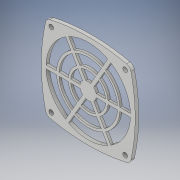
# Autodesk Inventor part: Speaker_Secure
Saved by Autodesk Inventor 2019.4 (Build 234330000, 330)
## iProperties
Created: 2020-04-12
Part Number: Speaker_Secure
Material: Типовые
Document SubType Name: Modeling
Designer: NoName
Density: 1 g/cm^3
Appearance: По умолчанию
Author: NoName
Autodesk Inventor part; units mm, degrees
ref_plane "YZ Plane" through (0, 0, 0) normal (1, 0, 0) x (0, 1, 0)
ref_plane "XZ Plane" through (0, 0, 0) normal (0, 1, 0) x (-1, 0, 0)
ref_plane "XY Plane" through (0, 0, 0) normal (0, 0, 1) x (1, 0, 0)
sketch "Эскиз1" plane through (0, 0, 0) normal (0, 0, 1) x (1, 0, 0)
  line L0 (-31.5, 31.5) -> (31.5, 31.5) construction
  line L1 (31.5, 31.5) -> (31.5, -31.5) construction
  line L2 (31.5, -31.5) -> (-31.5, -31.5) construction
  line L3 (-31.5, -31.5) -> (-31.5, 31.5) construction
  arc A0 (-32.5976, 36.378) -> (-36.378, 32.5976) centre (-31.5, 31.5) ccw
  line L4 (-40, 40) -> (40, 40) construction
  line L5 (40, 40) -> (40, -40) construction
  line L6 (40, -40) -> (-40, -40) construction
  line L7 (-40, -40) -> (-40, 40) construction
  arc A1 (-36.378, 32.5976) -> (-36.378, -32.5976) centre (108.5, 0) ccw
  line L8 (-40, 0) -> (40, 0)
  line L9 (0, 40) -> (0, -40)
  arc A2 (32.5976, 36.378) -> (-32.5976, 36.378) centre (0, -108.5) ccw
  arc A3 (36.378, 32.5976) -> (32.5976, 36.378) centre (31.5, 31.5) ccw
  arc A4 (-36.378, -32.5976) -> (-32.5976, -36.378) centre (-31.5, -31.5) ccw
  arc A5 (-32.5976, -36.378) -> (32.5976, -36.378) centre (0, 108.5) ccw
  arc A6 (36.378, -32.5976) -> (36.378, 32.5976) centre (-108.5, 0) ccw
  circle A7 centre (0, 0) radius 36
  circle A8 centre (-31.5, 31.5) radius 2
  circle A9 centre (31.5, 31.5) radius 2
  circle A10 centre (31.5, -31.5) radius 2
  circle A11 centre (-31.5, -31.5) radius 2
  arc A12 (32.5976, -36.378) -> (36.378, -32.5976) centre (31.5, -31.5) ccw
  point P0 (0, 31.5)
  point P1 (31.5, 0)
  dimension "d0" = 63
  dimension "d1" = 5
  dimension "d2" = 80
  dimension "d3" = 72
  dimension "d4" = 4
  constraints: 20 end point, 19 point on circle, 13 centre point, 7 coincident, 7 symmetric about line, 6 midpoint, 6 tangent, 4 parallel, 4 perpendicular, 3 equal radius, 3 horizontal, 2 horizontal alignment, 2 vertical alignment, 3 other
  measures "d0" distance of L0.start L0.end
  measures "d1" radius of A0
  measures "d2" distance of L4.start L4.end
  measures "d3" diameter of A7
  measures "d4" diameter of A9
extrude "Выдавливание1" add sketch "Эскиз1" along normal blind 3 contours A2 L9 A7 L8 A1 A0 | A2 A3 A6 L8 A7 L9 | L8 A7 L9 A5 A4 A1 | L8 A6 A12 A5 L9 A7
sketch "Эскиз2" plane through (0, 0, 3) normal (0, 0, 1) x (1, 0, 0)
  circle A0 centre (0, 0) radius 5
  circle A1 centre (0, 0) radius 7
  circle A2 centre (0, 0) radius 15
  circle A3 centre (0, 0) radius 17
  circle A4 centre (0, 0) radius 27
  circle A5 centre (0, 0) radius 25
  circle A6 centre (0, 0) radius 36 projected
  dimension "d7" = 2
  dimension "d8" = 2
  dimension "d9" = 2
  dimension "d10" = 10
  dimension "d11" = 30
  dimension "d12" = 50
  constraints: 6 centre point, 6 coincident
  measures "d7" radial gap between concentric circles of A1 A0
  measures "d8" radial gap between concentric circles of A3 A2
  measures "d9" radial gap between concentric circles of A4 A5
  measures "d10" diameter of A0
  measures "d11" diameter of A2
  measures "d12" diameter of A5
extrude "Выдавливание2" add sketch "Эскиз2" against normal blind 2 contours A1 | A3 | A4
sketch "Эскиз3" plane through (0, 0, 3) normal (0, 0, 1) x (1, 0, 0)
  line L0 (-39.9924, 1.5) -> (-6.8374, 1.5)
  line L1 (-6.8374, 1.5) -> (-6.8374, -1.5)
  line L2 (-6.8374, -1.5) -> (-39.9924, -1.5)
  line L3 (-39.9924, -1.5) -> (-39.9924, 1.5)
  circle A0 centre (0, 0) radius 7 projected
  arc A1 (-36.378, 32.5976) -> (-36.378, -32.5976) centre (108.5, 0) ccw projected
  dimension "d15" = 3
  constraints: 8 end point, 3 point on circle, 2 parallel, 1 horizontal, 1 perpendicular
  measures "d15" distance between parallel lines of L0 L2
extrude "Выдавливание3" add sketch "Эскиз3" against normal blind 2 contours L0 A0 L2 L3 | A0 L1 | L1 A0
pattern_circular "Круговой массив1" count 6 over 360 about axis through (0, 0, -10) along (0, 0, 1) of "Выдавливание3"
